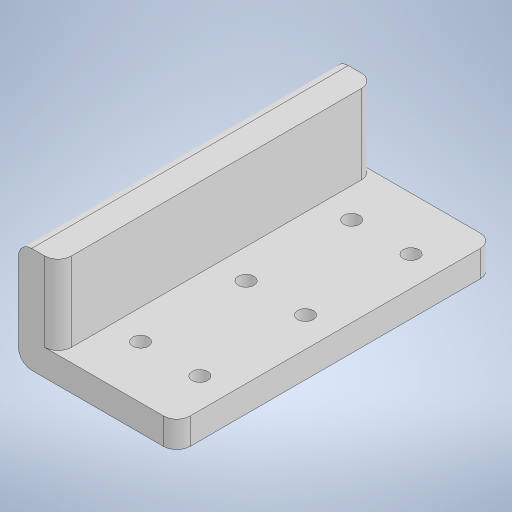
# Autodesk Inventor part: Arena Top Bracket
Saved by Autodesk Inventor 2023.4 (Build 274418000, 418)
## iProperties
Created: 2024-04-25
Part Number: Arena Top Bracket
Material: Generic
Document SubType Name: Modeling
Designer: Nathan Cai
Density: 1 g/cm^3
Appearance: Default
Author: Nathan Cai
Autodesk Inventor part; units mm, degrees
ref_plane "YZ Plane" through (0, 0, 0) normal (1, 0, 0) x (0, 1, 0)
ref_plane "XZ Plane" through (0, 0, 0) normal (0, 1, 0) x (-1, 0, 0)
ref_plane "XY Plane" through (0, 0, 0) normal (0, 0, 1) x (1, 0, 0)
sketch "Sketch1" plane through (0, 0, 0) normal (0, 0, 1) x (1, 0, 0)
  line L0 (0, 0) -> (9.525, 0)
  line L1 (9.525, 0) -> (9.525, 25.4)
  line L2 (9.525, 25.4) -> (0, 25.4)
  line L3 (0, 25.4) -> (0, 0)
  line L4 (0, 0) -> (38.1, 0)
  line L5 (38.1, 0) -> (38.1, 6.35)
  line L6 (38.1, 6.35) -> (0, 6.35)
  line L7 (0, 6.35) -> (0, 0)
  line L8 (9.525, 25.4) -> (12.7508, 25.4)
  line L9 (12.7508, 25.4) -> (12.7508, 0) construction
  line L10 (12.7508, 0) -> (9.525, 0)
  line L11 (9.525, 0) -> (9.525, 25.4)
  point P0 (9.525, 6.35)
  dimension "d0" = 9.525
  dimension "d1" = 25.4
  dimension "d2" = 38.1
  dimension "d3" = 6.35
  dimension "d4" = 3.2258
  constraints: 24 end point, 6 parallel, 3 horizontal, 3 perpendicular, 1 point on line
  measures "d0" distance of L2.end L1.end
  measures "d1" distance of L1.end L0.end
  measures "d2" distance of L6.end L5.end
  measures "d3" distance of L5.end L4.end
  measures "d4" distance of L9.end L10.end
extrude "Extrusion1" add sketch "Sketch1" along normal blind 76.2
sketch "Sketch2" plane through (9.525, 0, 0) normal (0, 1, 0) x (1, 0, 0)
  line L0 (28.575, -76.2) -> (0, -76.2) projected
  line L1 (14.2875, -76.2) -> (14.2875, 0) construction
  line L2 (28.575, 0) -> (0, 0) projected
  line L3 (28.575, 0) -> (28.575, -76.2) projected
  point P0 (-9.525, 0)
  point P1 (21.4312, -63.5)
  point P2 (21.4312, -38.1)
  point P3 (21.4312, -12.7)
  point P4 (7.1437, -63.5)
  point P5 (7.1437, -38.1)
  point P6 (7.1437, -12.7)
  dimension "d8" = 7.1437
  dimension "d9" = 14.2875
  dimension "d10" = 12.7
  dimension "d13" = 25.4
  dimension "d16" = 14.2875
  constraints: 2 end point, 2 midpoint, 1 horizontal, 1 vertical, 5 other
  measures "d8" distance from line of L3 point (21.431, -63.5)
  measures "d9" distance between parallel lines of L3 L1
  measures "d10" distance from line of L0 point (21.431, -63.5)
  measures "d13" distance of point (21.431, -63.5) point (21.431, -38.1)
  measures "d16" distance of point (21.431, -63.5) point (7.144, -63.5)
hole "Hole1" at (30.9563, 0, 63.5) at (30.9563, 0, 38.1) at (30.9563, 0, 12.7) at (16.6688, 0, 63.5) at (16.6688, 0, 38.1) at (16.6688, 0, 12.7) direction (0, 1, 0) diameter 3.81 end through all countersink diameter 7.0866 countersink angle 82 clearance for "Flat Head Machine Screw (82)" size "#6" standard "Ansi Unified Screw Threads"
fillet "Fillet1" radius 3.175 5 edges at (9.525, 15.875, 76.2) (9.525, 15.875, 0) (38.1, 3.175, 76.2) (38.1, 3.175, 0) (0, 0, 38.1)
fillet "Fillet2" radius 3.175 1 edges at (0, 25.4, 38.1)
equation "\"d8\" = 0.5 * d9"
equation "\"d16\" = d9"
body "Solid1"
